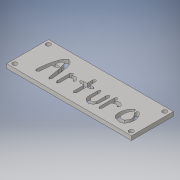
# Autodesk Inventor part: Name
Saved by Autodesk Inventor 2016 (Build 200138000, 138)
## iProperties
Created: 2016-09-23
Part Number: Name
Material: Generic
Document SubType Name: Sheet Metal
Designer: aesen
Density: 1 g/cm^3
Sheet Metal Rule: Default_mm
Appearance: Default
Author: aesen
Autodesk Inventor part; units mm, degrees
ref_plane "YZ Plane" through (0, 0, 0) normal (1, 0, 0) x (0, 1, 0)
ref_plane "XZ Plane" through (0, 0, 0) normal (0, 1, 0) x (-1, 0, 0)
ref_plane "XY Plane" through (0, 0, 0) normal (0, 0, 1) x (1, 0, 0)
sketch "Sketch2" plane through (0, 0, 0) normal (0, 0, 1) x (1, 0, 0)
  line L0 (0, 0) -> (300.1103, 0)
  line L1 (300.1103, 0) -> (300.1103, 100.8009)
  line L2 (300.1103, 100.8009) -> (0, 100.8009)
  line L3 (0, 100.8009) -> (0, 0)
  circle A0 centre (10, 90.343) radius 5.4183
  circle A1 centre (10, 10) radius 5.4183
  circle A2 centre (289.5422, 90.6602) radius 5.4183
  circle A3 centre (290.3474, 9.1425) radius 5.4183
  spline S0 degree 3 poles (47.0614, 25.4545) (47.528, 43.4805) (54.12, 78.9822) (64.9978, 83.5345) knots 0 0 0 0 1 1 1 1
  spline S1 degree 3 poles (64.9978, 83.5345) (83.6065, 81.6461) (82.7385, 43.7232) (85.9237, 25.4545) knots 0 0 0 0 1 1 1 1
  spline S2 degree 1 poles (55.389, 24.3869) (57.7378, 50.4375) knots 0 0 1 1
  spline S3 degree 2 poles (47.0614, 25.4545) (49.1255, 15.705) (55.389, 24.3869) knots 0 0 0 1 1 1
  spline S4 degree 1 poles (78.8772, 24.3869) (74.3931, 50.651) knots 0 0 1 1
  spline S5 degree 2 poles (78.8772, 24.3869) (83.5505, 13.6282) (85.9237, 25.4545) knots 0 0 0 1 1 1
  spline S6 degree 4 poles (59.019, 57.911) (58.4576, 61.6443) (68.1339, 91.1213) (71.7472, 59.0435) (72.6849, 58.1245) knots 0 0 0 0 0 1 1 1 1 1
  spline S7 degree 1 poles (96.1731, 25.0275) (96.1731, 55.7757) knots 0 0 1 1
  spline S8 degree 1 poles (103.4331, 25.0275) (103.4331, 44.0316) knots 0 0 1 1
  spline S9 degree 2 poles (103.4331, 44.0316) (109.8398, 52.1437) (116.2448, 44.0316) knots 0 0 0 1 1 1
  spline S10 degree 2 poles (103.4331, 52.3592) (109.9746, 59.5015) (116.2448, 51.7186) knots 0 0 0 1 1 1
  spline S11 degree 1 poles (103.4331, 52.3592) (103.4331, 55.7757) knots 0 0 1 1
  spline S12 degree 2 poles (103.4331, 55.7757) (100.4586, 63.4655) (96.1731, 55.7757) knots 0 0 0 1 1 1
  spline S13 degree 2 poles (116.2448, 51.7186) (121.8944, 46.0101) (116.2448, 44.0316) knots 0 0 0 1 1 1
  spline S14 degree 2 poles (96.1731, 25.0275) (100.5122, 14.8704) (103.4331, 25.0275) knots 0 0 0 1 1 1
  spline S15 degree 1 poles (137.5551, 24.3869) (137.5551, 48.0887) knots 0 0 1 1
  line L4 (144.815, 24.3869) -> (144.815, 48.0887)
  line L5 (144.815, 48.0887) -> (152.5021, 48.0887)
  line L6 (137.5551, 48.0887) -> (129.868, 48.0887)
  line L7 (137.5551, 55.7757) -> (129.868, 55.7757)
  line L8 (152.5021, 55.7757) -> (144.815, 55.7757)
  line L9 (144.815, 55.7757) -> (144.815, 69.6551)
  line L10 (137.5551, 55.7757) -> (137.5551, 69.6551)
  spline S16 degree 2 poles (137.5551, 24.3869) (140.9704, 16.0905) (144.815, 24.3869) knots 0 0 0 1 1 1
  spline S17 degree 2 poles (137.5551, 69.6551) (140.8285, 77.0951) (144.815, 69.6551) knots 0 0 0 1 1 1
  spline S18 degree 2 poles (152.5021, 55.7757) (161.0322, 52.5769) (152.5021, 48.0887) knots 0 0 0 1 1 1
  spline S19 degree 2 poles (129.868, 55.7757) (117.4806, 52.6672) (129.868, 48.0887) knots 0 0 0 1 1 1
  spline S20 degree 2 poles (165.9544, 27.1628) (181.1135, 4.9444) (193.2862, 27.1628) knots 0 0 0 1 1 1
  spline S21 degree 1 poles (165.9544, 27.1628) (165.9544, 52.359) knots 0 0 1 1
  spline S22 degree 1 poles (172.7874, 52.359) (172.7874, 30.1522) knots 0 0 1 1
  spline S23 degree 2 poles (172.7874, 30.1522) (181.8365, 16.2304) (186.8803, 29.7251) knots 0 0 0 1 1 1
  spline S24 degree 1 poles (186.8803, 29.7251) (186.5322, 52.344) knots 0 0 1 1
  spline S25 degree 1 poles (193.2862, 27.1628) (194.0062, 52.359) knots 0 0 1 1
  spline S26 degree 2 poles (165.9544, 52.359) (167.9027, 63.2961) (172.7874, 52.359) knots 0 0 0 1 1 1
  spline S27 degree 2 poles (194.0062, 52.359) (189.5472, 63.0062) (186.5322, 52.344) knots 0 0 0 1 1 1
  line L11 (200.8451, 22.6644) -> (200.8451, 58.3238)
  line L12 (207.6781, 22.6644) -> (207.6781, 43.3768)
  spline S28 degree 2 poles (200.8451, 22.6644) (204.6115, 13.7645) (207.6781, 22.6644) knots 0 0 0 1 1 1
  spline S29 degree 2 poles (207.6781, 43.3768) (215.6878, 50.9193) (222.6251, 43.3768) knots 0 0 0 1 1 1
  spline S30 degree 2 poles (207.6781, 51.7044) (215.1483, 58.6179) (222.6251, 52.9856) knots 0 0 0 1 1 1
  spline S31 degree 1 poles (207.6781, 51.7044) (207.6781, 58.3238) knots 0 0 1 1
  spline S32 degree 2 poles (200.8451, 58.3238) (204.6164, 65.9043) (207.6781, 58.3238) knots 0 0 0 1 1 1
  spline S33 degree 2 poles (222.6251, 52.9856) (229.0495, 47.1979) (222.6251, 43.3768) knots 0 0 0 1 1 1
  spline S34 degree 1 poles (59.019, 57.911) (67.7644, 58.3238) knots 0 0 1 1
  spline S35 degree 1 poles (57.7378, 50.4375) (66.4498, 51.7044) knots 0 0 1 1
  spline S36 degree 1 poles (72.6849, 58.1245) (74.3931, 50.651) knots 0 0 1 1
  spline S37 degree 2 poles (67.7644, 58.3238) (73.9281, 55.5594) (66.4498, 51.7044) knots 0 0 0 1 1 1
  spline S38 degree 3 poles (250.3077, 16.0597) (229.6641, 17.286) (235.0288, 49.9642) (248.7928, 59.6179) knots 0 0 0 0 1 1 1 1
  spline S39 degree 4 poles (250.3077, 16.0597) (265.1319, 9.4554) (277.4389, 34.9714) (273.4781, 48.5926) (254.3403, 65.288) (256.1147, 50.4005) knots 0 0 0 0 0 0.544263 1 1 1 1 1
  spline S40 degree 3 poles (248.7928, 50.4005) (245.7595, 44.1304) (238.6673, 17.9358) (259.1445, 24.3869) knots 0 0 0 0 1 1 1 1
  spline S41 degree 2 poles (259.1445, 24.3869) (271.6388, 36.6081) (256.1147, 50.4005) knots 0 0 0 1 1 1
  spline S42 degree 2 poles (248.7928, 59.6179) (255.8815, 56.0643) (248.7928, 50.4005) knots 0 0 0 1 1 1
  point P0 (50.0508, 50.4375)
  point P1 (57.7364, 75.2009)
  point P2 (76.3178, 75.1435)
  point P3 (82.9341, 50.4375)
  point P4 (50.0483, 20.3336)
  point P5 (82.9302, 19.2685)
  point P6 (62.1793, 68.1604)
  point P7 (66.4499, 71.5768)
  point P8 (70.5496, 65.8115)
  point P9 (109.8396, 48.0876)
  point P10 (109.8361, 55.7733)
  point P11 (100.2313, 59.6176)
  point P12 (119.033, 46.517)
  point P13 (100.2294, 19.9509)
  point P14 (141.048, 20.239)
  point P15 (140.9494, 73.3742)
  point P16 (156.7647, 52.3472)
  point P17 (123.6758, 52.3588)
  point P18 (180.6877, 16.0597)
  point P19 (181.2472, 23.0958)
  point P20 (168.5193, 57.821)
  point P21 (189.8394, 57.6769)
  point P22 (204.4763, 18.215)
  point P23 (215.5971, 47.1459)
  point P24 (215.3469, 55.4961)
  point P25 (204.4901, 62.1132)
  point P26 (225.828, 47.4324)
  point P27 (70.5492, 55.5893)
  point P28 (238.1887, 24.3868)
  point P29 (238.1887, 43.3767)
  point P30 (267.4763, 20.3332)
  point P31 (272.021, 36.2378)
  point P32 (267.4763, 50.4005)
  point P33 (259.1445, 58.3238)
  point P34 (245.763, 40.4941)
  point P35 (246.5206, 27.1626)
  point P36 (264.6991, 36.2378)
  point P37 (252.3275, 55.7757)
  dimension "d0" = 100.8009
  dimension "d1" = 300.1103
  dimension "d3" = 10.8366
  dimension "d4" = 10.8366
  dimension "d5" = 10.8366
  dimension "d6" = 10.8366
  dimension "d26" = 7.6871
  dimension "d27" = 8.541
  dimension "d28" = 8.3276
  dimension "d29" = 7.26
  dimension "d30" = 7.474
  dimension "d31" = 6.8329
  dimension "d32" = 7.26
  dimension "d33" = 8.3276
  dimension "d34" = 6.8329
  measures "d0" distance of L0.end L1.end
  measures "d1" distance of L1.end L2.end
  measures "d3" diameter of A0
  measures "d4" diameter of A1
  measures "d5" diameter of A2
  measures "d6" diameter of A3
  measures "d26" distance of point (57.738, 50.437) point (50.051, 50.437)
  measures "d27" horizontal distance of point (82.934, 50.437) point (74.393, 50.651)
  measures "d28" distance of point (103.433, 52.359) point (103.433, 44.032)
  measures "d29" distance of point (96.173, 25.027) point (103.433, 25.027)
  measures "d30" distance of point (194.006, 52.359) point (186.532, 52.344)
  measures "d31" distance of point (172.787, 52.359) point (165.954, 52.359)
  measures "d32" distance of L4.end L6.start
  measures "d33" distance of point (207.678, 51.704) L12.end
  measures "d34" distance of L11.start L12.start
extrude "Plate5" add sketch "Sketch2" along normal blind 10
equation "\"BendReliefDepth\" = 0.5 * Thickness"
equation "\"Thickness\" = 10"
body "Solid4"
